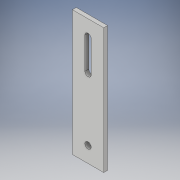
# Autodesk Inventor part: Slot Bumper attachment
Saved by Autodesk Inventor 2018 (Build 220112000, 112)
## iProperties
Created: 2019-01-26
Part Number: Slot Bumper attachment
Material: Generic
Document SubType Name: Modeling
Designer: s-2512711
Density: 1 g/cm^3
Appearance: Default
Author: s-2512711
Autodesk Inventor part; units mm, degrees
ref_plane "YZ Plane" through (0, 0, 0) normal (1, 0, 0) x (0, 1, 0)
ref_plane "XZ Plane" through (0, 0, 0) normal (0, 1, 0) x (-1, 0, 0)
ref_plane "XY Plane" through (0, 0, 0) normal (0, 0, 1) x (1, 0, 0)
sketch "Sketch1" plane through (0, 0, 0) normal (0, 0, 1) x (1, 0, 0)
  line L0 (0, 0) -> (25.4, 0)
  line L1 (25.4, 0) -> (25.4, 101.6)
  line L2 (25.4, 101.6) -> (0, 101.6)
  line L3 (0, 101.6) -> (0, 0)
  line L4 (12.7, 0) -> (12.7, 12.7) construction
  line L5 (12.7, 101.6) -> (12.7, 88.9) construction
  circle A0 centre (12.7, 12.7) radius 2.5797
  line L6 (12.7, 88.9) -> (12.7, 63.5) construction
  line L7 (10.1203, 88.9) -> (10.1203, 63.5)
  line L8 (15.2797, 63.5) -> (15.2797, 88.9)
  arc A1 (15.2797, 88.9) -> (10.1203, 88.9) centre (12.7, 88.9) ccw
  arc A2 (10.1203, 63.5) -> (15.2797, 63.5) centre (12.7, 63.5) ccw
  point P0 (12.7, 76.2)
  dimension "d0" = 25.4
  dimension "d1" = 101.6
  dimension "d2" = 12.7
  dimension "d3" = 12.7
  dimension "d7" = 25.4
  constraints: 20 end point, 4 point on circle, 4 tangent, 3 centre point, 3 midpoint, 3 parallel, 3 vertical, 1 coincident, 1 horizontal, 1 perpendicular
  measures "d0" distance of L2.end L1.end
  measures "d1" distance of L1.end L0.end
  measures "d2" distance of L4.start L4.end
  measures "d3" distance of L5.start L5.end
  measures "d7" distance of L5.end L6.end
extrude "Extrusion2" add sketch "Sketch1" along normal blind 3.175
body "Solid2"
